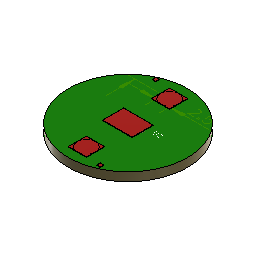
TOF Capsule v1 v8 (Autodesk Fusion 360 archive; units mm, degrees)
design "VL53L1X-TOF-Sensor"
part number: STAND-OFF
part number: FIDUCIALUFIDUCIAL
part number: 4.7uF
part number: OSHW-LOGOMINI
part number: VL53L1X
part number: 10k
part number: BM06B-SRSS-TBT(LF)(SN)
Autodesk Fusion 360 part; units mm, degrees
sketch "sketch 306" plane through (0, 0, 0) normal (0, 0, 1) x (1, 0, 0)
  circle A0 centre (11.43, 11.43) radius 10.925
extrude "Board" add sketch "sketch 306" along normal blind 1.57 makes body 1 in component "Board"
sketch "sketch 533" plane through (0, 0, 0) normal (0, 0, 1) x (1, 0, 0)
  line L0 (-1.651, -1.651) -> (1.651, -1.651)
  line L1 (1.651, -1.651) -> (1.651, 1.651)
  line L2 (1.651, 1.651) -> (-1.651, 1.651)
  line L3 (-1.651, 1.651) -> (-1.651, -1.651)
extrude "STAND-OFF" add sketch "sketch 533" along normal blind 0.1 separate body makes body 2 in component "STAND-OFF"
sketch "sketch 692" plane through (0, 0, 0) normal (0, 0, 1) x (1, 0, 0)
  line L0 (-0.3175, -0.3175) -> (0.3175, -0.3175)
  line L1 (0.3175, -0.3175) -> (0.3175, 0.3175)
  line L2 (0.3175, 0.3175) -> (-0.3175, 0.3175)
  line L3 (-0.3175, 0.3175) -> (-0.3175, -0.3175)
extrude "MICRO-FIDUCIAL" add sketch "sketch 692" along normal blind 0.1 separate body makes body 3 in component "MICRO-FIDUCIAL"
sketch "sketch 835" plane through (0, 0, 0) normal (0, 0, 1) x (1, 0, 0)
  line L0 (-0.838, -0.47) -> (0.83, -0.47)
  line L1 (0.83, -0.47) -> (0.83, 0.48)
  line L2 (0.83, 0.48) -> (-0.838, 0.48)
  line L3 (-0.838, 0.48) -> (-0.838, -0.47)
extrude "0603" add sketch "sketch 835" along normal blind 0.1 separate body makes body 4 in component "0603"
sketch "sketch 970" plane through (0, 0, 0) normal (0, 0, 1) x (1, 0, 0)
  line L0 (-1.233, -0.993) -> (1.237, -0.993)
  line L1 (1.237, -0.993) -> (1.237, 1.217)
  line L2 (1.237, 1.217) -> (-1.233, 1.217)
  line L3 (-1.233, 1.217) -> (-1.233, -0.993)
extrude "OSHW-LOGO-MINI" add sketch "sketch 970" along normal blind 0.1 separate body makes body 5 in component "OSHW-LOGO-MINI"
sketch "sketch 1105" plane through (0, 0, 0) normal (0, 0, 1) x (1, 0, 0)
  line L0 (-2.7, -1.941) -> (2.7, -1.941)
  line L1 (2.7, -1.941) -> (2.7, 1.9)
  line L2 (2.7, 1.9) -> (-2.7, 1.9)
  line L3 (-2.7, 1.9) -> (-2.7, -1.941)
extrude "VL53L1X" add sketch "sketch 1105" along normal blind 0.1 separate body makes body 6 in component "VL53L1X"
sketch "sketch 1248" plane through (0, 0, 0) normal (0, 0, 1) x (1, 0, 0)
  line L0 (-0.838, -0.47) -> (0.83, -0.47)
  line L1 (0.83, -0.47) -> (0.83, 0.48)
  line L2 (0.83, 0.48) -> (-0.838, 0.48)
  line L3 (-0.838, 0.48) -> (-0.838, -0.47)
extrude "0603'" add sketch "sketch 1248" along normal blind 0.1 separate body makes body 7 in component "0603 (1)"
sketch "sketch 1383" plane through (0, 0, 0) normal (0, 0, 1) x (1, 0, 0)
  line L0 (-4, -3.031) -> (4, -3.031)
  line L1 (4, -3.031) -> (4, 0.7)
  line L2 (4, 0.7) -> (-4, 0.7)
  line L3 (-4, 0.7) -> (-4, -3.031)
extrude "JST_BM06B-SRSS-TB(LF)(SN)" add sketch "sketch 1383" along normal blind 0.1 separate body makes body 8 in component "JST_BM06B-SRSS-TB(LF)(SN)"
sketch "sketch 398" plane through (0, 0, 0) normal (0, 0, 1) x (1, 0, 0)
  circle A0 centre (11.43, 19.05) radius 1.651
  circle A1 centre (11.43, 3.81) radius 1.651
extrude "Extrude2" cut sketch "sketch 398" along normal blind 1.57 bodies 1 in component "Board"
component "PCB Component" placed x (1, 0, 0) y (0, 1, 0) z (0, 0, 1) at (0, 0, 0)
component "Board" placed x (1, 0, 0) y (0, 1, 0) z (0, 0, 1) at (0, 0, 0) in component "PCB Component"
component "STAND-OFF" placed x (1, 0, 0) y (0, 1, 0) z (0, 0, 1) at (11.43, 19.05, 1.57) in component "PCB Component"
component "STAND-OFF" placed x (1, 0, 0) y (0, 1, 0) z (0, 0, 1) at (11.43, 3.81, 1.57) in component "PCB Component"
component "MICRO-FIDUCIAL" placed x (1, 0, 0) y (0, 1, 0) z (0, 0, 1) at (15.621, 2.159, 1.57) in component "PCB Component"
component "MICRO-FIDUCIAL" placed x (1, 0, 0) y (0, 1, 0) z (0, 0, 1) at (7.112, 20.828, 1.57) in component "PCB Component"
component "MICRO-FIDUCIAL" placed x (-1, 0, 0) y (0, 1, 0) z (0, 0, -1) at (7.112, 20.828, 0) in component "PCB Component"
component "MICRO-FIDUCIAL" placed x (-1, 0, 0) y (0, 1, 0) z (0, 0, -1) at (15.621, 2.159, 0) in component "PCB Component"
component "0603" placed x (1, 0, 0) y (0, -1, 0) z (0, 0, -1) at (13.97, 15.24, 0) in component "PCB Component"
component "0603" placed x (-1, 0, 0) y (0, 1, 0) z (0, 0, -1) at (13.97, 7.62, 0) in component "PCB Component"
component "OSHW-LOGO-MINI" placed x (-1, 0, 0) y (0, 1, 0) z (0, 0, -1) at (6.35, 3.81, 0) in component "PCB Component"
component "VL53L1X" placed x (1, 0, 0) y (0, 1, 0) z (0, 0, 1) at (11.43, 11.43, 1.57) in component "PCB Component"
component "0603 (1)" placed x (1, 0, 0) y (0, -1, 0) z (0, 0, -1) at (8.89, 15.24, 0) in component "PCB Component"
component "0603 (1)" placed x (1, 0, 0) y (0, -1, 0) z (0, 0, -1) at (10.16, 7.62, 0) in component "PCB Component"
component "JST_BM06B-SRSS-TB(LF)(SN)" placed x (0, -1, 0) y (-1, 0, 0) z (0, 0, -1) at (3.81, 11.43, 0) in component "PCB Component"
named bodies: "Board", "STAND-OFF", "MICRO-FIDUCIAL", "0603", "OSHW-LOGO-MINI", "VL53L1X", "JST_BM06B-SRSS-TB(LF)(SN)"
